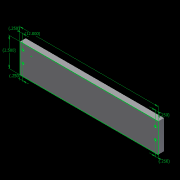
# Autodesk Inventor part: xcross1
Saved by Autodesk Inventor 2012 (Build 160160000, 160)
## iProperties
Created: 2011-09-28
Part Number: xcross1
Material: Default
Document SubType Name: Modeling
Designer: shane
Density: 1 g/cm^3
Author: shane
Autodesk Inventor part; units mm, degrees
ref_plane "YZ Plane" through (0, 0, 0) normal (1, 0, 0) x (0, 1, 0)
ref_plane "XZ Plane" through (0, 0, 0) normal (0, 1, 0) x (-1, 0, 0)
ref_plane "XY Plane" through (0, 0, 0) normal (0, 0, 1) x (1, 0, 0)
sketch "Sketch1" plane through (0, 0, 0) normal (0, 0, 1) x (1, 0, 0)
  line L0 (-24.9701, 15.4491) -> (279.8299, 15.4491)
  line L1 (279.8299, 15.4491) -> (279.8299, -48.0509)
  line L2 (279.8299, -48.0509) -> (-24.9701, -48.0509)
  line L3 (-24.9701, -48.0509) -> (-24.9701, 15.4491)
  point P0 (0, 0)
  dimension "d0" = 304.8
  dimension "d1" = 63.5
  constraints: 8 end point, 2 parallel, 1 horizontal, 1 perpendicular
  measures "d0" distance of L0.start L0.end
  measures "d1" distance of L2.end L0.start
extrude "Extrusion1" add sketch "Sketch1" along normal blind 12.7
hole "Hole1" at (-18.6201, 2.7491, 12.7) direction (0, 0, -1) diameter 4.826 end through all
hole "Hole2" at (-18.6201, -22.6509, 12.7) direction (0, 0, -1) diameter 4.826 end through all
hole "Hole3" at (273.4799, 2.7491, 12.7) direction (0, 0, -1) diameter 4.826 end through all
hole "Hole4" at (273.4799, -22.6509, 12.7) direction (0, 0, -1) diameter 4.826 end through all
sketch "Sketch2" plane through (0, 0, 12.7) normal (0, 0, 1) x (1, 0, 0)
  circle A0 centre (273.4799, -22.6509) radius 2.413 projected
  circle A1 centre (273.4799, 2.7491) radius 2.413 projected
  circle A2 centre (-18.6201, -22.6509) radius 2.413 projected
  circle A3 centre (-18.6201, 2.7491) radius 2.413 projected
  line L0 (279.8299, 15.4491) -> (279.8299, -48.0509) projected
  line L1 (-24.9701, 15.4491) -> (279.8299, 15.4491) projected
  line L2 (-24.9701, -48.0509) -> (-24.9701, 15.4491) projected
  line L3 (279.8299, -48.0509) -> (-24.9701, -48.0509) projected
  point P0 (0, 0)
  dimension "d40" = 304.8
  dimension "d41" = 63.5
  dimension "d42" = 6.35
  dimension "d43" = 6.35
  dimension "d44" = 6.35
  dimension "d45" = 6.35
  measures "d40" distance of L1.start L0.start
  measures "d41" distance of L2.start L1.start
  measures "d42" distance from line of L2 A3.centre
  measures "d43" distance from line of L2 A2.centre
  measures "d44" distance from line of L0 A1.centre
  measures "d45" distance from line of L0 A0.centre
sketch "Sketch3" plane through (0, 0, 12.7) normal (0, 0, 1) x (1, 0, 0)
  circle A0 centre (273.4799, -22.6509) radius 2.413 projected
  circle A1 centre (273.4799, 2.7491) radius 2.413 projected
  circle A2 centre (-18.6201, -22.6509) radius 2.413 projected
  circle A3 centre (-18.6201, 2.7491) radius 2.413 projected
  line L0 (279.8299, 15.4491) -> (279.8299, -48.0509) projected
  line L1 (-24.9701, 15.4491) -> (279.8299, 15.4491) projected
  line L2 (-24.9701, -48.0509) -> (-24.9701, 15.4491) projected
  line L3 (279.8299, -48.0509) -> (-24.9701, -48.0509) projected
  point P0 (0, 0)
body "Solid1"
